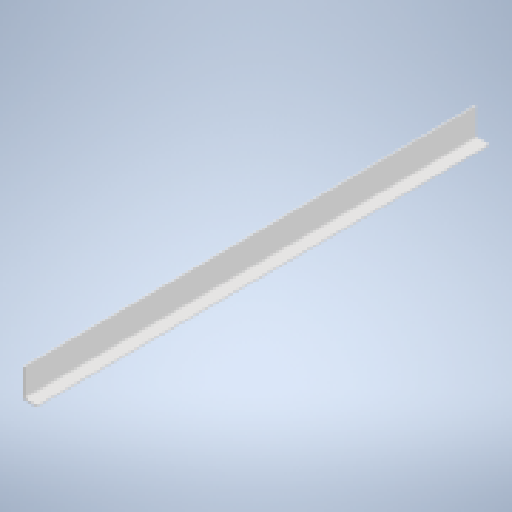
# Autodesk Inventor part: L_Channel
Saved by Autodesk Inventor 2023 (Build 270158000, 158)
## iProperties
Created: 2022-05-10
Part Number: L_Channel
Material: Generic
Document SubType Name: Modeling
Designer: a laptop
Density: 1 g/cm^3
Appearance: Default
Author: a laptop
Autodesk Inventor part; units mm, degrees
ref_plane "YZ Plane" through (0, 0, 0) normal (1, 0, 0) x (0, 1, 0)
ref_plane "XZ Plane" through (0, 0, 0) normal (0, 1, 0) x (-1, 0, 0)
ref_plane "XY Plane" through (0, 0, 0) normal (0, 0, 1) x (1, 0, 0)
sketch "Sketch1" plane through (0, 0, 0) normal (0, 0, 1) x (1, 0, 0)
  line L0 (0, 3.175) -> (0, 76.2)
  line L1 (0, 76.2) -> (3.175, 76.2)
  line L2 (3.175, 76.2) -> (3.175, 6.35)
  line L3 (6.35, 3.175) -> (38.1, 3.175)
  line L4 (38.1, 3.175) -> (38.1, 0)
  line L5 (38.1, 0) -> (3.175, 0)
  arc A0 (3.175, 6.35) -> (6.35, 3.175) centre (6.35, 6.35) ccw
  arc A1 (0, 3.175) -> (3.175, 0) centre (3.175, 3.175) ccw
  point P0 (0, 0)
  dimension "d0" = 3.175
  dimension "d1" = 38.1
  dimension "d2" = 76.2
  dimension "d3" = 3.175
  constraints: 12 end point, 6 perpendicular, 4 point on circle, 4 tangent, 2 centre point, 2 point on line, 1 equal radius, 1 vertical
  measures "d0" distance of L0.end L1.end
  measures "d1" distance of L4.end point (0, 0)
  measures "d2" distance of point (0, 0) L0.end
  measures "d3" radius of A0
extrude "Extrusion1" add sketch "Sketch1" along normal blind 1219.2
body "Solid1"
